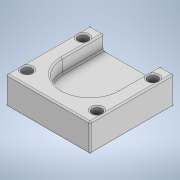
# Autodesk Inventor part: Base
Saved by Autodesk Inventor 2022 (Build 260153000, 153)
## iProperties
Created: 2022-03-31
Part Number: Base
Material: Generic
Document SubType Name: Modeling
Designer: thoms
Density: 1 g/cm^3
Appearance: Default
Author: thoms
Autodesk Inventor part; units mm, degrees
ref_plane "YZ Plane" through (0, 0, 0) normal (1, 0, 0) x (0, 1, 0)
ref_plane "XZ Plane" through (0, 0, 0) normal (0, 1, 0) x (-1, 0, 0)
ref_plane "XY Plane" through (0, 0, 0) normal (0, 0, 1) x (1, 0, 0)
sketch "Sketch1" plane through (0, 0, 0) normal (0, 1, 0) x (-1, 0, 0)
  line L0 (15, 15) -> (-15, 15)
  line L1 (-15, 15) -> (-15, -15)
  line L2 (-15, -15) -> (15, -15)
  line L3 (15, -15) -> (15, 15)
  point P0 (0, 0)
  dimension "d0" = 30
  dimension "d1" = 30
  dimension "d2" = 15
  dimension "d3" = 15
  constraints: 8 end point, 2 parallel, 1 horizontal, 1 perpendicular
  measures "d0" distance of L1.end L2.end
  measures "d1" distance of L0.end L1.end
  measures "d2" distance from line of point (0, 0) L1
  measures "d3" distance from line of point (0, 0) L0
extrude "Extrusion1" add sketch "Sketch1" against normal blind 10
sketch "Sketch2" plane through (0, 0, 0) normal (0, 1, 0) x (1, 0, 0)
  arc A0 (-10, 0) -> (10, 0) centre (0, 0) ccw
  line L0 (-10, 0) -> (-10, 15)
  line L1 (-15, 15) -> (15, 15) projected
  line L2 (10, 0) -> (10, 15)
  line L3 (-10, 15) -> (10, 15)
  dimension "d6" = 20
  constraints: 6 end point, 2 point on circle, 2 point on line, 1 centre point, 1 coincident, 1 collinear, 1 perpendicular, 1 tangent, 1 vertical
  measures "d6" diameter of A0
extrude "Extrusion2" cut sketch "Sketch2" against normal blind 5
sketch "Sketch3" plane through (0, 0, 0) normal (0, 1, 0) x (1, 0, 0)
  circle A0 centre (-12.5, 10) radius 1.5
  line L0 (-10, 15) -> (-15, 15) projected
  line L1 (-15, 15) -> (-15, -15) projected
  circle A1 centre (-12.5, -10) radius 1.5
  line L2 (-15, -15) -> (15, -15) projected
  circle A2 centre (12.5, -10) radius 1.5
  line L3 (15, -15) -> (15, 15) projected
  circle A3 centre (12.5, 10) radius 1.5
  line L4 (15, 15) -> (10, 15) projected
  point P0 (0, 0)
  dimension "d9" = 3
  dimension "d10" = 5
  dimension "d11" = 2.5
  dimension "d12" = 3
  dimension "d13" = 2.5
  dimension "d14" = 5
  dimension "d15" = 5
  dimension "d16" = 2.5
  dimension "d17" = 3
  dimension "d18" = 2.5
  dimension "d19" = 5
  dimension "d20" = 3
  constraints: 4 centre point
  measures "d9" diameter of A0
  measures "d10" distance from line of L0 A0.centre
  measures "d11" distance from line of L1 A0.centre
  measures "d12" diameter of A1
  measures "d13" distance from line of L1 A1.centre
  measures "d14" distance from line of L2 A1.centre
  measures "d15" distance from line of L2 A2.centre
  measures "d16" distance from line of L3 A2.centre
  measures "d17" diameter of A2
  measures "d18" distance from line of L3 A3.centre
  measures "d19" distance from line of L4 A3.centre
  measures "d20" diameter of A3
extrude "Extrusion3" cut sketch "Sketch3" against normal blind 5
sketch "Sketch4" plane through (0, 0, 0) normal (0, 1, 0) x (1, 0, 0)
  circle A0 centre (-12.5, -10) radius 1.5 projected
  circle A1 centre (-12.5, -10) radius 1.75
  circle A2 centre (-12.5, 10) radius 1.5 projected
  circle A3 centre (-12.5, 10) radius 1.75
  circle A4 centre (12.5, -10) radius 1.5 projected
  circle A5 centre (12.5, -10) radius 1.75
  circle A6 centre (12.5, 10) radius 1.75
  point P0 (0, 0)
  dimension "d23" = 3.5
  dimension "d24" = 3.5
  dimension "d25" = 3.5
  dimension "d27" = 3.5
  constraints: 4 centre point, 3 coincident
  measures "d23" diameter of A1
  measures "d24" diameter of A3
  measures "d25" diameter of A5
  measures "d27" diameter of A6
extrude "Extrusion4" cut sketch "Sketch4" against normal blind 4 contours A0 | A1 | A2 | A3 | A4 | A5 | A6
fillet "Fillet1" radius 0.5 30 edges at (-14, -4, -10) (11, -4, -10) (11, -4, 10) (10.75, 0, 10) (10.75, 0, -10) (-14.25, 0, -10) (-14, -4, 10) (-14.25, 0, 10) (-10, 0, -7.5) (10, 0, -7.5) (0, 0, 10) (0, -5, 10) (10, -5, -7.5) (-10, -5, -7.5) (0, -5, -15) (-12.5, 0, -15) (-15, 0, 0) (0, 0, 15) (15, 0, 0) (12.5, 0, -15) (15, -5, -15) (15, -5, 15) (-15, -5, 15) (-15, -5, -15) (-10, -2.5, -15) (10, -2.5, -15) (-15, -10, 0) (0, -10, 15) (15, -10, 0) (0, -10, -15)
body "Solid1"
